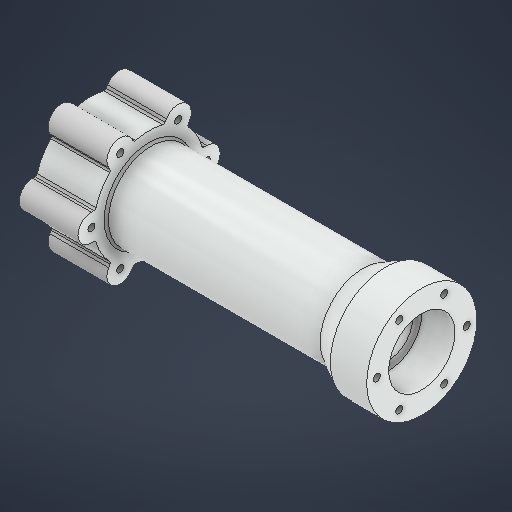
# Autodesk Inventor part: Body
Saved by Autodesk Inventor 2026.1 (Build 301233020, 233B)
## iProperties
Created: 2025-10-11
Part Number: Body
Material: Generic
Document SubType Name: Modeling
Designer: Alexander
Density: 1 g/cm^3
Appearance: Default
Author: Alexander
Autodesk Inventor part; units mm, degrees
ref_plane "YZ Plane" through (0, 0, 0) normal (1, 0, 0) x (0, 1, 0)
ref_plane "XZ Plane" through (0, 0, 0) normal (0, 1, 0) x (-1, 0, 0)
ref_plane "XY Plane" through (0, 0, 0) normal (0, 0, 1) x (1, 0, 0)
sketch "Sketch1" plane through (0, 0, 0) normal (0, 1, 0) x (-1, 0, 0)
  line L0 (100, 40) -> (-100, 40)
  line L1 (-100, 40) -> (-121, 51.5)
  line L2 (-121, 51.5) -> (-155, 51.5)
  line L3 (-155, 51.5) -> (-155, 31)
  line L4 (-155, 31) -> (-100, 31)
  line L5 (-100, 31) -> (-100, 34)
  line L6 (-100, 34) -> (100, 34)
  line L7 (100, 34) -> (100, 31)
  line L8 (100, 31) -> (155, 31)
  line L9 (155, 31) -> (155, 51.5)
  line L10 (155, 51.5) -> (100, 51.5)
  line L11 (100, 51.5) -> (100, 40)
  line L12 (217, 0) -> (-217, 0) projected
  point P0 (0, 0)
  point P1 (0, 40)
  dimension "d0" = 0
  dimension "d1" = 200
  dimension "d2" = 34
  dimension "d3" = 51.5
  dimension "d4" = 55
  dimension "d5" = 40
  dimension "d6" = 20.5
  dimension "d7" = 55
  dimension "d8" = 3
  dimension "d9" = 200
  dimension "d10" = 3
  dimension "d11" = 55
  dimension "d12" = 20.5
  dimension "d13" = 55
  dimension "d14" = 31
  constraints: 24 end point, 3 perpendicular, 2 horizontal, 2 parallel, 2 point on line, 1 midpoint, 1 vertical
  measures "d0" horizontal distance of point (0, 0) point (0, 40)
  measures "d1" distance of L0.start L0.end
  measures "d2" distance of L1.end L2.end
  measures "d3" distance from line of point (0, 0) L2
  measures "d4" horizontal distance of L0.end L2.end
  measures "d5" distance from line of point (0, 0) L0
  measures "d6" distance of L2.end L3.end
  measures "d7" distance of L3.end L4.end
  measures "d8" distance of L4.end L5.end
  measures "d9" distance of L5.end L6.end
  measures "d10" distance of L6.end L7.end
  measures "d11" distance of L7.end L8.end
  measures "d12" distance of L8.end L9.end
  measures "d13" distance of L9.end L10.end
  measures "d14" distance from line of point (0, 0) L8
revolve "Revolution1" add sketch "Sketch1" angle 360 about axis through (-10, 0, 0) along (1, 0, 0)
sketch "Sketch2" plane through (155, 0, 0) normal (1, 0, 0) x (0, 0, -1)
  point P0 (0, 0)
  point P1 (42, 0)
  dimension "d16" = 42
  measures "d16" distance of point (0, 0) point (42, 0)
hole "Hole1" at (155, 0, -42) direction (-1, 0, 0) diameter 6.647 depth 22.2 tip angle 118 thread size "M8x1.25" class "6H" standard "ISO Metric profile"
pattern_circular "Circular Pattern1" count 6 over 360 about axis through (-10, 0, 0) along (1, 0, 0) of "Hole1"
sketch "Sketch3" plane through (-155, 0, 0) normal (-1, 0, 0) x (0, 0, 1)
  circle A0 centre (54, 0) radius 12.5
  circle A1 centre (27, 46.7654) radius 12.5
  circle A2 centre (-27, 46.7654) radius 12.5
  circle A3 centre (-54, 0) radius 12.5
  circle A4 centre (-27, -46.7654) radius 12.5
  circle A5 centre (27, -46.7654) radius 12.5
  line L0 (49.5676, 60.8535) -> (-26.8685, -71.5377)
  line L1 (23.5368, 65.7668) -> (-47.874, -57.9201)
  line L2 (-21.0315, 61.4276) -> (45.2687, -53.4077)
  line L3 (23.2328, -65.2403) -> (-46.41, 55.3845)
  line L4 (-72.6311, 12.5) -> (88.6525, 12.5)
  line L5 (81.3558, -12.5) -> (-74.1802, -12.5)
  circle A6 centre (0, 0) radius 51.5
  point P0 (-14.1547, 49.5166)
  point P1 (-16.1747, 53.0154)
  point P2 (-37.8253, 40.5154)
  point P3 (-35.8053, 37.0166)
  point P4 (-49.96, 12.5)
  point P5 (-54, 12.5)
  point P6 (-54, -12.5)
  point P7 (-49.96, -12.5)
  point P8 (-35.8053, -37.0166)
  point P9 (-37.8253, -40.5154)
  point P10 (-16.1747, -53.0154)
  point P11 (-14.1547, -49.5166)
  point P12 (14.1547, -49.5166)
  point P13 (16.1747, -53.0154)
  point P14 (37.8253, -40.5154)
  point P15 (35.8053, -37.0166)
  point P16 (49.96, -12.5)
  point P17 (54, -12.5)
  point P18 (54, 12.5)
  point P19 (49.96, 12.5)
  point P20 (35.8053, 37.0166)
  point P21 (37.8253, 40.5154)
  point P22 (16.1747, 53.0154)
  point P23 (14.1547, 49.5166)
  dimension "d27" = 54
  dimension "d28" = 25
  dimension "d31" = 360
  constraints: 12 end point, 12 tangent, 7 centre point, 2 coincident, 1 horizontal, 13 other
  measures "d27" distance of point (0, 0) point (54, 0)
  measures "d28" diameter of A0
extrude "Extrusion1" add sketch "Sketch3" against normal blind 55 contours A0 A6 | A0 A6 L4 | L5 A6 A0 | A6 A1 L0 | L2 A5 A6 | A1 A6 | A5 A6 | A6 L1 A1 | A5 L3 A6 | A6 A2 L2 | L0 A4 A6 | A2 A6 | L3 A2 A6 | A6 A3 L4 | A4 A6 | A6 A4 L1 | L5 A3 A6 | A3 A6 picked at (56.0357, 3.1385) picked at (28.5319, 48.6266) picked at (28.5319, -48.6266) picked at (-27.7482, 49.0658) picked at (-27.7482, -49.0658) picked at (-56.3663, -0.5022)
sketch "Sketch4" plane through (-100, 0, -54) normal (1, 0, 0) x (0, 0, -1)
  arc A0 (0, -12.5) -> (0, 12.5) centre (0, 0) ccw projected
  point P0 (-54, 0)
  constraints: 1 coincident
hole "Hole2" at (-100, 0, -54) at (-100, 0, -54) direction (-1, 0, 0) diameter 6.647 end through all thread size "M8x1.25" class "6H" standard "ISO Metric profile"
pattern_circular "Circular Pattern2" count 6 over 360 about axis through (-10, 0, 0) along (1, 0, 0) of "Hole2"
fillet "Fillet1" radius 2 13 edges at (-127.5, 37.0166, 35.8053) (-100, 0, -40) (-127.5, 12.5, 49.96) (-127.5, -12.5, 49.96) (-127.5, -37.0166, 35.8053) (-127.5, -49.5166, -14.1547) (-127.5, -49.5166, 14.1547) (-127.5, -37.0166, -35.8053) (-127.5, -12.5, -49.96) (-127.5, 37.0166, -35.8053) (-127.5, 12.5, -49.96) (-127.5, 49.5166, 14.1547) (-127.5, 49.5166, -14.1547)
sketch "Sketch5" plane through (0, 0, 0) normal (0, 1, 0) x (-1, 0, 0)
  line L0 (-100, -34) -> (100, -34) projected
  line L1 (-100, -34) -> (-124, -34)
  line L2 (-124, -34) -> (-124, -22.5)
  line L3 (-124, -22.5) -> (-100, -22.5)
  line L4 (-100, -22.5) -> (-100, -34)
  line L5 (143.8, 0) -> (-162.8, 0) projected
  point P0 (0, 0)
  dimension "d47" = 24
  dimension "d49" = 22.5
  dimension "d50" = 100
  constraints: 8 end point, 2 parallel, 1 horizontal, 1 perpendicular, 1 point on line
  measures "d47" distance between parallel lines of L2 L4
  measures "d49" distance from line of point (0, 0) L3
  measures "d50" distance from line of point (0, 0) L4
revolve "Revolution2" add sketch "Sketch5" angle 360 about axis through (-10, 0, 0) along (1, 0, 0)
body "Solid1"
